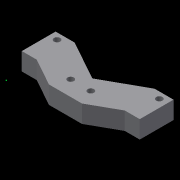
# Autodesk Inventor part: AX_XY
Saved by Autodesk Inventor 2016 (Build 200138000, 138)
## iProperties
Created: 2017-08-22
Part Number: AX_XY
Material: Generic
Document SubType Name: Modeling
Designer: ludwi
Density: 1 g/cm^3
Appearance: Default
Author: ludwi
Autodesk Inventor part; units mm, degrees
ref_plane "YZ Plane" through (0, 0, 0) normal (1, 0, 0) x (0, 1, 0)
ref_plane "XZ Plane" through (0, 0, 0) normal (0, 1, 0) x (-1, 0, 0)
ref_plane "XY Plane" through (0, 0, 0) normal (0, 0, 1) x (1, 0, 0)
sketch "Sketch1" plane through (0, 0, 0) normal (0, 0, 1) x (1, 0, 0)
  line L0 (-58, -50) -> (-58, 50) construction
  line L1 (-58, -50) -> (58, -50) construction
  line L2 (58, 50) -> (58, -50) construction
  line L3 (58, 50) -> (-58, 50) construction
  line L4 (-48.8, -35) -> (-48.8, -43.5) construction
  arc A0 (-55.2, -43.5) -> (-48.8, -43.5) centre (-52, -43.5) ccw construction
  line L5 (-55.2, -43.5) -> (-55.2, -35) construction
  arc A1 (-48.8, -35) -> (-55.2, -35) centre (-52, -35) ccw construction
  line L6 (55.2, -35) -> (55.2, -43.5) construction
  arc A2 (48.8, -43.5) -> (55.2, -43.5) centre (52, -43.5) ccw construction
  line L7 (48.8, -43.5) -> (48.8, -35) construction
  arc A3 (55.2, -35) -> (48.8, -35) centre (52, -35) ccw construction
  circle A4 centre (10.25, -35) radius 3.2 construction
  circle A5 centre (-10.25, -35) radius 3.2 construction
  circle A6 centre (-10.25, 35) radius 3.2 construction
  circle A7 centre (10.25, 35) radius 3.2 construction
  line L8 (-55.2, 35) -> (-55.2, 43.5) construction
  arc A8 (-48.8, 43.5) -> (-55.2, 43.5) centre (-52, 43.5) ccw construction
  line L9 (-48.8, 43.5) -> (-48.8, 35) construction
  arc A9 (-55.2, 35) -> (-48.8, 35) centre (-52, 35) ccw construction
  circle A10 centre (-52, 7.125) radius 3.2 construction
  line L10 (-7.05, -7.125) -> (-7.05, -15.625) construction
  arc A11 (-13.45, -15.625) -> (-7.05, -15.625) centre (-10.25, -15.625) ccw construction
  line L11 (-13.45, -15.625) -> (-13.45, -7.125) construction
  arc A12 (-7.05, -7.125) -> (-13.45, -7.125) centre (-10.25, -7.125) ccw construction
  circle A13 centre (52, -7.125) radius 3.2 construction
  circle A14 centre (-52, -7.125) radius 3.2 construction
  line L12 (13.45, -7.125) -> (13.45, -15.625) construction
  arc A15 (7.05, -15.625) -> (13.45, -15.625) centre (10.25, -15.625) ccw construction
  line L13 (7.05, -15.625) -> (7.05, -7.125) construction
  arc A16 (13.45, -7.125) -> (7.05, -7.125) centre (10.25, -7.125) ccw construction
  circle A17 centre (52, 7.125) radius 3.2 construction
  line L14 (13.45, 15.625) -> (13.45, 7.125) construction
  arc A18 (7.05, 7.125) -> (13.45, 7.125) centre (10.25, 7.125) ccw construction
  line L15 (7.05, 7.125) -> (7.05, 15.625) construction
  arc A19 (13.45, 15.625) -> (7.05, 15.625) centre (10.25, 15.625) ccw construction
  line L16 (55.2, 43.5) -> (55.2, 35) construction
  arc A20 (48.8, 35) -> (55.2, 35) centre (52, 35) ccw construction
  line L17 (48.8, 35) -> (48.8, 43.5) construction
  arc A21 (55.2, 43.5) -> (48.8, 43.5) centre (52, 43.5) ccw construction
  line L18 (-7.05, 15.625) -> (-7.05, 7.125) construction
  arc A22 (-13.45, 7.125) -> (-7.05, 7.125) centre (-10.25, 7.125) ccw construction
  line L19 (-13.45, 7.125) -> (-13.45, 15.625) construction
  arc A23 (-7.05, 15.625) -> (-13.45, 15.625) centre (-10.25, 15.625) ccw construction
  line L20 (60, 50) -> (58, 50) construction
  line L21 (58, 50) -> (58, -50) construction
  line L22 (58, -50) -> (60, -50) construction
  line L23 (60, -50) -> (60, 50) construction
  line L24 (-60, -50) -> (-58, -50) construction
  line L25 (-58, -50) -> (-58, 50) construction
  line L26 (-58, 50) -> (-60, 50) construction
  line L27 (-60, 50) -> (-60, -50) construction
  line L28 (-60, 50) -> (-60, 15.625)
  line L29 (-60, 15.625) -> (-44.7827, 15.625)
  line L30 (-44.7827, 15.625) -> (-16.7505, 0)
  line L31 (-60, 50) -> (-40.7335, 50)
  line L32 (-40.7335, 50) -> (0, 27.4416)
  line L33 (0, 27.4416) -> (0, 0)
  line L34 (0, 0) -> (-16.7505, 0)
  circle A24 centre (-52, 43.5) radius 3.2
  circle A25 centre (-10.25, 15.625) radius 3.2
  line L35 (0, 50) -> (0, 0) construction
  line L36 (60, 50) -> (60, 15.625)
  line L37 (60, 15.625) -> (44.7827, 15.625)
  line L38 (44.7827, 15.625) -> (16.7505, 0)
  line L39 (60, 50) -> (40.7335, 50)
  line L40 (40.7335, 50) -> (0, 27.4416)
  line L41 (0, 0) -> (16.7505, 0)
  circle A26 centre (52, 43.5) radius 3.2
  circle A27 centre (10.25, 15.625) radius 3.2
  constraints: 28 end point, 6 symmetric about line, 2 centre point, 2 coincident, 2 horizontal alignment, 2 perpendicular, 2 point on line, 1 horizontal, 1 midpoint, 1 vertical, 6 other
extrude "Extrusion1" add sketch "Sketch1" along normal blind 18
chamfer "Chamfer1" distance 28 angle 45 1 edges at (0, 27.4416, 9)
sketch "Sketch2" plane through (-60, 15.625, 0) normal (-1, 0, 0) x (0, 0, 1)
  line L0 (2, -65.625) -> (2, 34.375) projected
  line L1 (2, -65.625) -> (18, -65.625) projected
  line L2 (18, -53.625) -> (18, -65.625) projected
  arc A0 (18, -37.625) -> (18, -53.625) centre (18, -45.625) ccw projected
  line L3 (18, -27.625) -> (18, -37.625) projected
  arc A1 (18, -3.625) -> (18, -27.625) centre (18, -15.625) ccw projected
  line L4 (18, 6.375) -> (18, -3.625) projected
  arc A2 (18, 22.375) -> (18, 6.375) centre (18, 14.375) ccw projected
  line L5 (18, 34.375) -> (18, 22.375) projected
  line L6 (2, 34.375) -> (18, 34.375) projected
  line L7 (18, 34.375) -> (18, 0) projected
  point P0 (0, -15.625)
extrude "Extrusion2" cut sketch "Sketch2" against normal through all contours L7 A2
sketch "Sketch3" plane through (0, 0, 18) normal (0, 0, 1) x (1, 0, 0)
  circle A0 centre (10.25, 15.625) radius 3.2 projected
  circle A1 centre (-10.25, 15.625) radius 3.2 projected
  line L0 (60, 22) -> (-60, 22) projected
  line L1 (-60, 22) -> (-60, 15.625) projected
  line L2 (-60, 15.625) -> (-44.7827, 15.625) projected
  line L3 (-44.7827, 15.625) -> (-16.7505, 0) projected
  line L4 (-16.7505, 0) -> (16.7505, 0) projected
  line L5 (16.7505, 0) -> (44.7827, 15.625) projected
  line L6 (44.7827, 15.625) -> (60, 15.625) projected
  line L7 (60, 15.625) -> (60, 22) projected
  line L8 (30.7666, 7.8125) -> (-30.7666, 7.8125)
  point P0 (0, 0)
  constraints: 2 end point, 2 midpoint, 1 horizontal
extrude "Extrusion3" cut sketch "Sketch3" against normal through all contours L5 L4 L3 L8
chamfer "Chamfer2" distance 2 angle 45 6 edges at (-60, 32.8125, 0) (60, 32.8125, 0) (37.7747, 11.7188, 0) (-37.7747, 11.7188, 0) (-32.6141, 45.5034, 0) (32.6141, 45.5034, 0)
body "Solid1"
